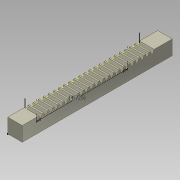
# Autodesk Inventor part: RAM
Saved by Autodesk Inventor 2012 SP2 (Build 160219200, 219)
## iProperties
Shininess: 64.0
Length Units: 11272
Angle Units: 11279
Time Units: 11290
Mass Units: 11286
Length Display Precision: 3
Angle Display Precision: 2
Compacted: True
Part Number: RAM
Document SubType Name: Modeling
Created: 2003-11-19
Designer: Autodesk, Inc.
Manufacturer: Standard
Standards Organization: Custom
Mass: 509.763 g
Surface Area: 178.528 cm^2
Volume: 65.0208 cm^3
Density: 7.84 g/cm^3
Material: Steel, High Strength Low Alloy
Density: 0.0
Volumn: 0.0
Area: 0.0
PropertySet Name: Model Information
Control State: 0
Master: False
Checked Out: False
Author: Autodesk, Inc.
Autodesk Inventor part; units mm, degrees
sketch "Sketch1" plane through (0, 0, 0) normal (0, 0, 1) x (1, 0, 0)
  line L0 (0, 0) -> (19.05, 0)
  line L1 (19.05, 0) -> (19.05, 19.05)
  line L2 (19.05, 19.05) -> (0, 19.05)
  line L3 (0, 19.05) -> (0, 0)
  dimension "d0" = 19.05
  dimension "d1" = 19.05
  constraints: 8 end point, 2 parallel, 1 horizontal, 1 perpendicular
  measures "d0" distance of L0.start L0.end
  measures "d1" distance of L0.end L1.end
extrude "Extrusion1" add sketch "Sketch1" along normal blind 196.85
sketch "Sketch2" plane through (19.05, 0, 0) normal (1, 0, 0) x (0, 0, -1)
  line L0 (0, 0) -> (0, 19.05) projected
  line L1 (0, 19.05) -> (-196.85, 19.05) projected
  line L2 (-196.85, 19.05) -> (-196.85, 0) projected
  line L3 (0, 0) -> (-196.85, 0) projected
  line L4 (-168.1851, 19.05) -> (-166.4005, 19.05)
  line L5 (-166.4005, 19.05) -> (-164.7392, 14.4856)
  line L6 (-168.1851, 19.05) -> (-169.8464, 14.4856)
  line L7 (-167.2928, 19.05) -> (-167.2928, 27.5407) construction
  line L8 (-130.1446, 19.8229) -> (-130.1446, 4.5609) construction
  line L9 (-173.4311, 16.9342) -> (-94.8151, 16.9342) construction
  line L10 (-163.1967, 14.4856) -> (-161.5354, 19.05)
  line L11 (-161.5354, 19.05) -> (-159.7508, 19.05)
  line L12 (-159.7508, 19.05) -> (-158.0895, 14.4856)
  line L13 (-164.7392, 14.4856) -> (-163.1967, 14.4856)
  line L14 (-158.0895, 14.4856) -> (-24.9935, 14.4856) construction
  line L15 (-160.6431, 19.05) -> (-160.6431, 25.2679) construction
  line L16 (-169.8464, 14.4856) -> (-171.3889, 14.4856)
  line L17 (-171.3889, 14.4856) -> (-173.0502, 19.05)
  line L18 (-156.5419, 14.4856) -> (-154.8806, 19.05)
  line L19 (-154.8806, 19.05) -> (-153.096, 19.05)
  line L20 (-153.096, 19.05) -> (-151.4347, 14.4856)
  line L21 (-149.8871, 14.4856) -> (-148.2258, 19.05)
  line L22 (-148.2258, 19.05) -> (-146.4412, 19.05)
  line L23 (-146.4412, 19.05) -> (-144.7799, 14.4856)
  line L24 (-143.2323, 14.4856) -> (-141.571, 19.05)
  line L25 (-141.571, 19.05) -> (-139.7864, 19.05)
  line L26 (-139.7864, 19.05) -> (-138.1251, 14.4856)
  line L27 (-136.5775, 14.4856) -> (-134.9162, 19.05)
  line L28 (-134.9162, 19.05) -> (-133.1316, 19.05)
  line L29 (-133.1316, 19.05) -> (-131.4703, 14.4856)
  line L30 (-129.9227, 14.4856) -> (-128.2614, 19.05)
  line L31 (-128.2614, 19.05) -> (-126.4768, 19.05)
  line L32 (-126.4768, 19.05) -> (-124.8155, 14.4856)
  line L33 (-123.2679, 14.4856) -> (-121.6066, 19.05)
  line L34 (-121.6066, 19.05) -> (-119.822, 19.05)
  line L35 (-119.822, 19.05) -> (-118.1607, 14.4856)
  line L36 (-116.6131, 14.4856) -> (-114.9518, 19.05)
  line L37 (-114.9518, 19.05) -> (-113.1672, 19.05)
  line L38 (-113.1672, 19.05) -> (-111.5059, 14.4856)
  line L39 (-109.9583, 14.4856) -> (-108.297, 19.05)
  line L40 (-108.297, 19.05) -> (-106.5124, 19.05)
  line L41 (-106.5124, 19.05) -> (-104.8511, 14.4856)
  line L42 (-103.3035, 14.4856) -> (-101.6422, 19.05)
  line L43 (-101.6422, 19.05) -> (-99.8576, 19.05)
  line L44 (-99.8576, 19.05) -> (-98.1963, 14.4856)
  line L45 (-96.6487, 14.4856) -> (-94.9874, 19.05)
  line L46 (-94.9874, 19.05) -> (-93.2028, 19.05)
  line L47 (-93.2028, 19.05) -> (-91.5415, 14.4856)
  line L48 (-89.9939, 14.4856) -> (-88.3326, 19.05)
  line L49 (-88.3326, 19.05) -> (-86.548, 19.05)
  line L50 (-86.548, 19.05) -> (-84.8867, 14.4856)
  line L51 (-83.3391, 14.4856) -> (-81.6778, 19.05)
  line L52 (-81.6778, 19.05) -> (-79.8932, 19.05)
  line L53 (-79.8932, 19.05) -> (-78.2319, 14.4856)
  line L54 (-76.6843, 14.4856) -> (-75.023, 19.05)
  line L55 (-75.023, 19.05) -> (-73.2384, 19.05)
  line L56 (-73.2384, 19.05) -> (-71.5771, 14.4856)
  line L57 (-70.0295, 14.4856) -> (-68.3682, 19.05)
  line L58 (-68.3682, 19.05) -> (-66.5836, 19.05)
  line L59 (-66.5836, 19.05) -> (-64.9223, 14.4856)
  line L60 (-63.3747, 14.4856) -> (-61.7134, 19.05)
  line L61 (-61.7134, 19.05) -> (-59.9288, 19.05)
  line L62 (-59.9288, 19.05) -> (-58.2675, 14.4856)
  line L63 (-56.7199, 14.4856) -> (-55.0586, 19.05)
  line L64 (-55.0586, 19.05) -> (-53.274, 19.05)
  line L65 (-53.274, 19.05) -> (-51.6127, 14.4856)
  line L66 (-50.0651, 14.4856) -> (-48.4038, 19.05)
  line L67 (-48.4038, 19.05) -> (-46.6192, 19.05)
  line L68 (-46.6192, 19.05) -> (-44.9579, 14.4856)
  line L69 (-43.4103, 14.4856) -> (-41.749, 19.05)
  line L70 (-41.749, 19.05) -> (-39.9644, 19.05)
  line L71 (-39.9644, 19.05) -> (-38.3031, 14.4856)
  line L72 (-36.7555, 14.4856) -> (-35.0942, 19.05)
  line L73 (-35.0942, 19.05) -> (-33.3096, 19.05)
  line L74 (-33.3096, 19.05) -> (-31.6483, 14.4856)
  line L75 (-30.1007, 14.4856) -> (-28.4394, 19.05)
  line L76 (-28.4394, 19.05) -> (-26.6548, 19.05) construction
  line L77 (-26.6548, 19.05) -> (-24.9935, 14.4856) construction
  line L78 (-158.0895, 14.4856) -> (-156.5419, 14.4856)
  line L79 (-151.4347, 14.4856) -> (-149.8871, 14.4856)
  line L80 (-144.7799, 14.4856) -> (-143.2323, 14.4856)
  line L81 (-138.1251, 14.4856) -> (-136.5775, 14.4856)
  line L82 (-131.4703, 14.4856) -> (-129.9227, 14.4856)
  line L83 (-124.5031, 14.4856) -> (-123.2679, 14.4856)
  line L84 (-117.895, 14.4856) -> (-116.6131, 14.4856)
  line L85 (-124.5031, 14.4856) -> (-124.8155, 14.4856)
  line L86 (-117.895, 14.4856) -> (-118.1607, 14.4856)
  line L87 (-111.5059, 14.4856) -> (-109.9583, 14.4856)
  line L88 (-104.8511, 14.4856) -> (-103.3035, 14.4856)
  line L89 (-98.1963, 14.4856) -> (-96.6487, 14.4856)
  line L90 (-91.5415, 14.4856) -> (-89.9939, 14.4856)
  line L91 (-84.8867, 14.4856) -> (-83.3391, 14.4856)
  line L92 (-78.2319, 14.4856) -> (-76.6843, 14.4856)
  line L93 (-71.5771, 14.4856) -> (-70.0295, 14.4856)
  line L94 (-64.9223, 14.4856) -> (-63.3747, 14.4856)
  line L95 (-58.2675, 14.4856) -> (-56.7199, 14.4856)
  line L96 (-51.6127, 14.4856) -> (-50.0651, 14.4856)
  line L97 (-44.9579, 14.4856) -> (-43.4103, 14.4856)
  line L98 (-30.1007, 14.4856) -> (-31.6483, 14.4856)
  line L99 (-38.3031, 14.4856) -> (-36.7555, 14.4856)
  line L100 (-28.4394, 19.05) -> (0, 19.05)
  line L101 (0, 0) -> (0, 19.05)
  line L102 (0, 0) -> (-196.85, 0)
  line L103 (-196.85, 0) -> (-196.85, 19.05)
  line L104 (-196.85, 19.05) -> (-173.0502, 19.05)
  point P0 (-168.9552, 16.9342)
  point P1 (-165.6304, 16.9342)
  point P2 (-162.3055, 16.9342)
  point P3 (-158.9807, 16.9342)
  point P4 (-172.2801, 16.9342)
  point P5 (-153.9883, 19.05)
  point P6 (-155.6507, 16.9342)
  point P7 (-152.3259, 16.9342)
  point P8 (-147.3335, 19.05)
  point P9 (-148.9959, 16.9342)
  point P10 (-145.6711, 16.9342)
  point P11 (-140.6787, 19.05)
  point P12 (-142.3411, 16.9342)
  point P13 (-139.0163, 16.9342)
  point P14 (-134.0239, 19.05)
  point P15 (-135.6863, 16.9342)
  point P16 (-132.3615, 16.9342)
  point P17 (-127.3691, 19.05)
  point P18 (-129.0315, 16.9342)
  point P19 (-125.7067, 16.9342)
  point P20 (-120.7143, 19.05)
  point P21 (-122.3767, 16.9342)
  point P22 (-119.0519, 16.9342)
  point P23 (-114.0595, 19.05)
  point P24 (-115.7219, 16.9342)
  point P25 (-112.3971, 16.9342)
  point P26 (-107.4047, 19.05)
  point P27 (-109.0671, 16.9342)
  point P28 (-105.7423, 16.9342)
  point P29 (-100.7499, 19.05)
  point P30 (-102.4123, 16.9342)
  point P31 (-99.0875, 16.9342)
  point P32 (-94.0951, 19.05)
  point P33 (-95.7575, 16.9342)
  point P34 (-92.4327, 16.9342)
  point P35 (-87.4403, 19.05)
  point P36 (-89.1027, 16.9342)
  point P37 (-85.7779, 16.9342)
  point P38 (-80.7855, 19.05)
  point P39 (-82.4479, 16.9342)
  point P40 (-79.1231, 16.9342)
  point P41 (-74.1307, 19.05)
  point P42 (-75.7931, 16.9342)
  point P43 (-72.4683, 16.9342)
  point P44 (-67.4759, 19.05)
  point P45 (-69.1383, 16.9342)
  point P46 (-65.8135, 16.9342)
  point P47 (-60.8211, 19.05)
  point P48 (-62.4835, 16.9342)
  point P49 (-59.1587, 16.9342)
  point P50 (-54.1663, 19.05)
  point P51 (-55.8287, 16.9342)
  point P52 (-52.5039, 16.9342)
  point P53 (-47.5115, 19.05)
  point P54 (-49.1739, 16.9342)
  point P55 (-45.8491, 16.9342)
  point P56 (-40.8567, 19.05)
  point P57 (-42.5191, 16.9342)
  point P58 (-39.1943, 16.9342)
  point P59 (-34.2019, 19.05)
  point P60 (-35.8643, 16.9342)
  point P61 (-32.5395, 16.9342)
  point P62 (-27.5471, 19.05)
  point P63 (-29.2095, 16.9342)
  point P64 (-25.8847, 16.9342)
  dimension "d5" = 2.1158
  dimension "d6" = 20
  dimension "d7" = 20
  dimension "d11" = 6.6497
  dimension "d12" = 3.3249
  dimension "d13" = 3.3249
  dimension "d14" = 3.3249
  dimension "d15" = 23.7998
  dimension "d16" = 2.4486
  dimension "d19" = 6.6548
  constraints: 201 end point, 53 point on line, 27 collinear, 10 parallel, 3 perpendicular, 2 midpoint, 1 coincident, 1 horizontal, 200 other
  measures "d5" distance between parallel lines of L9 L4
  measures "d6" angle of L7 L6
  measures "d7" angle of L5 L7
  measures "d11" distance between parallel lines of L15 L7
  measures "d12" distance of point (-165.63, 16.934) point (-168.955, 16.934)
  measures "d13" distance of point (-158.981, 16.934) point (-162.306, 16.934)
  measures "d14" distance of point (-168.955, 16.934) point (-172.28, 16.934)
  measures "d15" distance from line of L2 L17.end
  measures "d16" distance between parallel lines of L16 L9
  measures "d19" distance of L10.start L18.start
extrude "Extrusion2" cut sketch "Sketch2" against normal through all contours L3 L2 L1 L17 L16 L6 L5 L13 L10 L12 L78 L18 L20 L79 L21 L23 L80 L24 L26 L81 L27 L29 L82 L30 L32 L85 L83 L33 L35 L86 L84 L36 L38 L87 L39 L41 L88 L42 L44 L89 L45 L47 L90 L48 L50 L91 L51 L53 L92 L54 L56 L93 L57 L59 L94 L60 L62 L95 L63 L65 L96 L66 L68 L97 L69 L71 L99 L72 L74 L98 L75 L0 keep common part
sketch "Sketch5" plane through (19.05, 0, 196.85) normal (1, 0, 0) x (0, 0, -1)
  line L0 (126.8205, 14.4856) -> (128.4818, 19.05) projected
  line L1 (125.2729, 14.4856) -> (126.8205, 14.4856) projected
  line L2 (123.6116, 19.05) -> (125.2729, 14.4856) projected
  line L3 (123.6116, 19.05) -> (121.827, 19.05) projected
  line L4 (120.1657, 14.4856) -> (121.827, 19.05) projected
  line L5 (118.6181, 14.4856) -> (120.1657, 14.4856) projected
  line L6 (116.9568, 19.05) -> (118.6181, 14.4856) projected
  line L7 (116.9568, 19.05) -> (115.1722, 19.05) projected
  line L8 (113.5109, 14.4856) -> (115.1722, 19.05) projected
  line L9 (111.9633, 14.4856) -> (113.5109, 14.4856) projected
  line L10 (110.302, 19.05) -> (111.9633, 14.4856) projected
  line L11 (110.302, 19.05) -> (108.5174, 19.05) projected
  line L12 (106.8561, 14.4856) -> (108.5174, 19.05) projected
  line L13 (105.3085, 14.4856) -> (106.8561, 14.4856) projected
  line L14 (103.6472, 19.05) -> (105.3085, 14.4856) projected
  line L15 (103.6472, 19.05) -> (101.8626, 19.05) projected
  line L16 (100.2013, 14.4856) -> (101.8626, 19.05) projected
  line L17 (98.6537, 14.4856) -> (100.2013, 14.4856) projected
  line L18 (96.9924, 19.05) -> (98.6537, 14.4856) projected
  line L19 (96.9924, 19.05) -> (95.2078, 19.05) projected
  line L20 (93.5465, 14.4856) -> (95.2078, 19.05) projected
  line L21 (91.9989, 14.4856) -> (93.5465, 14.4856) projected
  line L22 (90.3376, 19.05) -> (91.9989, 14.4856) projected
  line L23 (90.3376, 19.05) -> (88.553, 19.05) projected
  line L24 (86.8917, 14.4856) -> (88.553, 19.05) projected
  line L25 (85.3441, 14.4856) -> (86.8917, 14.4856) projected
  line L26 (83.6828, 19.05) -> (85.3441, 14.4856) projected
  line L27 (83.6828, 19.05) -> (81.8982, 19.05) projected
  line L28 (80.2369, 14.4856) -> (81.8982, 19.05) projected
  line L29 (78.6893, 14.4856) -> (80.2369, 14.4856) projected
  line L30 (77.028, 19.05) -> (78.6893, 14.4856) projected
  line L31 (77.028, 19.05) -> (75.2434, 19.05) projected
  line L32 (73.5821, 14.4856) -> (75.2434, 19.05) projected
  line L33 (72.0345, 14.4856) -> (73.5821, 14.4856) projected
  line L34 (70.3732, 19.05) -> (72.0345, 14.4856) projected
  line L35 (70.3732, 19.05) -> (68.5886, 19.05) projected
  line L36 (66.9273, 14.4856) -> (68.5886, 19.05) projected
  line L37 (65.3797, 14.4856) -> (66.9273, 14.4856) projected
  line L38 (63.7184, 19.05) -> (65.3797, 14.4856) projected
  line L39 (63.7184, 19.05) -> (61.9338, 19.05) projected
  line L40 (60.2725, 14.4856) -> (61.9338, 19.05) projected
  line L41 (58.7249, 14.4856) -> (60.2725, 14.4856) projected
  line L42 (57.0636, 19.05) -> (58.7249, 14.4856) projected
  line L43 (57.0636, 19.05) -> (55.279, 19.05) projected
  line L44 (53.6177, 14.4856) -> (55.279, 19.05) projected
  line L45 (52.0701, 14.4856) -> (53.6177, 14.4856) projected
  line L46 (50.4088, 19.05) -> (52.0701, 14.4856) projected
  line L47 (50.4088, 19.05) -> (48.6242, 19.05) projected
  line L48 (46.9629, 14.4856) -> (48.6242, 19.05) projected
  line L49 (45.4153, 14.4856) -> (46.9629, 14.4856) projected
  line L50 (43.754, 19.05) -> (45.4153, 14.4856) projected
  line L51 (43.754, 19.05) -> (41.9694, 19.05) projected
  line L52 (40.3081, 14.4856) -> (41.9694, 19.05) projected
  line L53 (38.7605, 14.4856) -> (40.3081, 14.4856) projected
  line L54 (37.0992, 19.05) -> (38.7605, 14.4856) projected
  line L55 (37.0992, 19.05) -> (35.3146, 19.05) projected
  line L56 (33.6533, 14.4856) -> (35.3146, 19.05) projected
  line L57 (32.1108, 14.4856) -> (33.6533, 14.4856) projected
  line L58 (30.4495, 19.05) -> (32.1108, 14.4856) projected
  line L59 (30.4495, 19.05) -> (28.6649, 19.05) projected
  line L60 (27.0036, 14.4856) -> (28.6649, 19.05) projected
  line L61 (25.4611, 14.4856) -> (27.0036, 14.4856) projected
  line L62 (23.7998, 19.05) -> (25.4611, 14.4856) projected
  line L63 (23.7998, 19.05) -> (0, 19.05) projected
  line L64 (0, 19.05) -> (0, 0) projected
  line L65 (196.85, 0) -> (0, 0) projected
  line L66 (196.85, 0) -> (196.85, 19.05) projected
  line L67 (196.85, 19.05) -> (168.4106, 19.05) projected
  line L68 (166.7493, 14.4856) -> (168.4106, 19.05) projected
  line L69 (165.2017, 14.4856) -> (166.7493, 14.4856) projected
  line L70 (163.5404, 19.05) -> (165.2017, 14.4856) projected
  line L71 (163.5404, 19.05) -> (161.7558, 19.05) projected
  line L72 (160.0945, 14.4856) -> (161.7558, 19.05) projected
  line L73 (158.5469, 14.4856) -> (160.0945, 14.4856) projected
  line L74 (156.8856, 19.05) -> (158.5469, 14.4856) projected
  line L75 (156.8856, 19.05) -> (155.101, 19.05) projected
  line L76 (153.4397, 14.4856) -> (155.101, 19.05) projected
  line L77 (151.8921, 14.4856) -> (153.4397, 14.4856) projected
  line L78 (150.2308, 19.05) -> (151.8921, 14.4856) projected
  line L79 (150.2308, 19.05) -> (148.4462, 19.05) projected
  line L80 (146.7849, 14.4856) -> (148.4462, 19.05) projected
  line L81 (145.2373, 14.4856) -> (146.7849, 14.4856) projected
  line L82 (143.576, 19.05) -> (145.2373, 14.4856) projected
  line L83 (143.576, 19.05) -> (141.7914, 19.05) projected
  line L84 (140.1301, 14.4856) -> (141.7914, 19.05) projected
  line L85 (138.5825, 14.4856) -> (140.1301, 14.4856) projected
  line L86 (136.9212, 19.05) -> (138.5825, 14.4856) projected
  line L87 (136.9212, 19.05) -> (135.1366, 19.05) projected
  line L88 (133.4753, 14.4856) -> (135.1366, 19.05) projected
  line L89 (131.9277, 14.4856) -> (133.4753, 14.4856) projected
  line L90 (130.2664, 19.05) -> (131.9277, 14.4856) projected
  line L91 (130.2664, 19.05) -> (128.4818, 19.05) projected
  line L92 (168.4106, 19.05) -> (170.3156, 19.05)
  line L93 (170.3156, 19.05) -> (171.9769, 14.4856)
  line L94 (171.9769, 14.4856) -> (173.5263, 14.4856)
  line L95 (173.5263, 14.4856) -> (175.1876, 19.05)
  line L96 (170.3156, 19.05) -> (175.1876, 19.05)
  dimension "d26" = 1.5494
  dimension "d27" = 1.905
  constraints: 10 end point, 3 parallel, 2 collinear, 2 point on line
  measures "d26" distance of L93.end L94.end
  measures "d27" distance of L67.end L92.end
extrude "Extrusion3" cut sketch "Sketch5" against normal blind 25.4 contours L67 L95 L94 L93
ref_plane "Work Plane1" through (9.525, 0, 196.85) normal (1, 0, 0) x (0, 0, -1)
ref_plane "Work Plane2" through (0, 0, 98.425) normal (0, 0, -1) x (-1, 0, 0)
sketch "Sketch6" plane through (0, 0, 0) normal (-1, 0, 0) x (0, 0, 1)
  line L0 (28.4394, 19.05) -> (30.1007, 14.4856) projected
  line L1 (30.1007, 14.4856) -> (28.4394, 19.05) projected
  line L2 (22.4325, 16.9342) -> (172.2801, 16.9342)
  dimension "d1" = 19.05
  dimension "d30" = 149.8476
  constraints: 2 end point, 2 other
  measures "d30" distance of L2.start L2.end
ref_plane "Work Plane3" through (0, 16.9342, 172.2801) normal (0, 1, 0) x (-1, 0, 0)
sketch "Sketch7" plane through (0, 0, 0) normal (-1, 0, 0) x (0, 0, 1)
  line L0 (169.8464, 14.4856) -> (171.3889, 14.4856) projected
  line L1 (169.8464, 14.4856) -> (169.8464, 42.6146)
  line L2 (168.1851, 19.05) -> (169.8464, 14.4856) projected
  point P0 (0, 0)
  dimension "d1" = 19.05
  constraints: 2 end point
ref_plane "Work Plane4" through (0, 16.9342, 172.2801) normal (0, 0, 1) x (1, 0, 0)
ref_plane "Work Plane5" through (0, 16.7678, 22.4931) normal (0, 0, -1) x (-1, 0, 0)
sketch "Sketch8" plane through (0, 0, 0) normal (-1, 0, 0) x (0, 0, 1)
  line L0 (172.2801, 28.8683) -> (172.2801, 16.9342)
  line L1 (157.4011, 16.9342) -> (157.4011, 0)
  line L2 (37.3775, 0) -> (37.3775, 16.9342)
  line L3 (172.2801, 28.8683) -> (172.2801, 16.9342)
  line L4 (22.4931, 28.8683) -> (22.4931, 16.9342)
  line L5 (22.4931, 16.9342) -> (157.4011, 16.9342)
  line L6 (157.4011, 16.9342) -> (172.2801, 16.9342)
  dimension "d1" = 19.05
  dimension "d32" = 120.0236
  constraints: 14 end point, 3 coincident
  measures "d32" distance between parallel lines of L1 L2
sketch "Sketch9" plane through (19.05, 0, 196.85) normal (1, 0, 0) x (0, 0, -1)
  line L0 (24.5699, 28.8683) -> (24.5699, 16.9342) projected
  line L1 (39.4489, 16.9342) -> (39.4489, 0) projected
  line L2 (159.4725, 0) -> (159.4725, 16.9342) projected
  line L3 (174.3569, 28.8683) -> (174.3569, 16.9342) projected
  line L4 (24.5699, 16.9342) -> (174.3569, 16.9342)
  point P0 (196.85, 0)
  dimension "d1" = 19.05
  dimension "d33" = 120.0236
  constraints: 4 coincident, 2 end point
  measures "d33" distance between parallel lines of L2 L1
sketch "Sketch10" plane through (19.05, 0, 196.85) normal (1, 0, 0) x (0, 0, -1)
  line L0 (152.5443, 11.2798) -> (167.7772, 11.2798) construction
  line L1 (167.7772, 11.2798) -> (167.7772, 4.5864) construction
  line L2 (167.7772, 4.5864) -> (152.5443, 4.5864) construction
  line L3 (152.5443, 4.5864) -> (152.5443, 11.2798) construction
  point P0 (196.85, 0)
  dimension "d1" = 19.05
  constraints: 2 other
ref_plane "Work Plane7" through (19.05, 16.9342, 37.3775) normal (0, 0, -1) x (-1, 0, 0)
equation "\"d13\" = d12"
equation "\"d14\" = d12"
body "Solid1"
